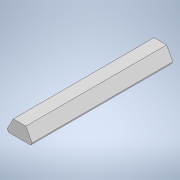
# Autodesk Inventor part: dishHolderArm
Saved by Autodesk Inventor 2022.2 (Build 262287010, 287A)
## iProperties
Created: 2021-09-26
Part Number: dishHolderArm
Material: Generic
Document SubType Name: Modeling
Designer: yiunf
Density: 1 g/cm^3
Appearance: Default
Author: yiunf
## iProperties of the stored document dishHolderArm_3DPrint.ipt
Created: 2021-09-26
Part Number: dishHolderArm_3DPrint
Material: Generic
Document SubType Name: Modeling
Designer: yiunf
Density: 1 g/cm^3
Appearance: Default
Author: yiunf
Autodesk Inventor part; units mm, degrees
ref_plane "YZ Plane" through (0, 0, 0) normal (1, 0, 0) x (0, 1, 0)
ref_plane "XZ Plane" through (0, 0, 0) normal (0, 1, 0) x (-1, 0, 0)
ref_plane "XY Plane" through (0, 0, 0) normal (0, 0, 1) x (1, 0, 0)
sketch "Sketch1" plane through (0, 0, 0) normal (0, 0, 1) x (1, 0, 0)
  line L0 (0, 0) -> (-4.9, 0)
  line L1 (-4.9, 0) -> (4.9, 0)
  line L2 (0, 0) -> (0, 5)
  line L3 (0, 5) -> (-2.5, 5)
  line L4 (-2.5, 5) -> (-4.9, 0)
  line L5 (0, 5) -> (2.5, 5)
  line L6 (2.5, 5) -> (4.9, 0)
  line L7 (0, 0) -> (0, 4)
  line L8 (0, 4) -> (-2.5, 4)
  line L9 (-2.5, 4) -> (-4.9, 0)
  line L10 (0, 4) -> (2.5, 4)
  line L11 (2.5, 4) -> (4.9, 0)
  line L12 (0, 4) -> (0, 5)
  line L13 (0, 4.5) -> (-2.5, 4.5)
  line L14 (-2.5, 4.5) -> (-4.9, 0)
  line L15 (0, 4.5) -> (2.5, 4.5)
  line L16 (2.5, 4.5) -> (4.9, 0)
  line L17 (-4.9, 0) -> (-2.2333, 5)
  line L18 (4.9, 0) -> (2.2333, 5)
  dimension "d0" = 4.9
  dimension "d1" = 9.8
  dimension "d5" = 5
  dimension "d6" = 2.5
  dimension "d7" = 2.5
  dimension "d33" = 4
  constraints: 38 end point, 7 point on line, 3 horizontal, 2 perpendicular, 1 collinear, 1 midpoint, 1 symmetric about line, 1 vertical
  measures "d0" distance of L0.start L0.end
  measures "d1" distance of L0.end L1.end
  measures "d5" distance of L0.start L2.end
  measures "d6" distance of L2.end L3.end
  measures "d7" distance of L2.end L5.end
  measures "d33" distance of L0.start L7.end
extrude "Extrusion1" add sketch "Sketch1" along normal blind 50 contours L2 L10 L11 L1 | L0 L9 L8 L2 | L14 L13 L2 L8 L9 | L11 L10 L2 L15 L16 | L17 L3 L2 L13 | L15 L2 L5 L18
sketch "Sketch2" plane through (0, 0, 50) normal (0, 0, 1) x (1, 0, 0)
  line L0 (0, 5) -> (0, -65)
  circle A0 centre (0, -30) radius 35
  line L1 (-4.9, 0) -> (4.9, 0) projected
  line L2 (4.9, 0) -> (18.0278, 0)
  arc A1 (18.0278, 0) -> (2.5, 5) centre (2.5, -21.6111) ccw
  line L3 (4.9, 0) -> (0, 0)
  line L4 (2.5, 5) -> (0, 5)
  line L5 (-4.9, 0) -> (-18.0278, 0)
  arc A2 (-2.5, 5) -> (-18.0278, 0) centre (-2.5, -21.6111) ccw
  circle A3 centre (0, -30) radius 37.5
  line L6 (2.5, 6.0566) -> (32.476, -11.25)
  line L7 (32.476, -11.25) -> (32.476, -48.75)
  line L8 (32.476, -48.75) -> (0, -67.5)
  line L9 (0, -67.5) -> (-32.476, -48.75)
  line L10 (-32.476, -48.75) -> (-32.476, -11.25)
  line L11 (-32.476, -11.25) -> (-2.5, 6.0566)
  arc A4 (2.5, 6.0566) -> (-2.5, 6.0566) centre (0, 1.7265) ccw
  line L12 (-4.9, 0) -> (-12.9904, 0)
  line L13 (4.9, 0) -> (12.9904, 0)
  line L14 (4.9, 0) -> (-4.9, 0)
  circle A5 centre (0, -30) radius 30
  line L15 (-17.488, -2.5967) -> (0, -30)
  line L16 (0, -30) -> (17.488, -2.5967)
  circle A6 centre (0, -30) radius 32.508
  line L17 (0, -30) -> (-32.476, -11.25)
  line L18 (0, -30) -> (32.476, -11.25)
  arc A7 (-29.976, -9.8066) -> (-32.476, -14.1368) centre (-27.476, -14.1368) ccw
  arc A8 (-32.476, -45.8632) -> (-29.976, -50.1934) centre (-27.476, -45.8632) ccw
  arc A9 (-2.5, -66.0566) -> (2.5, -66.0566) centre (0, -61.7265) ccw
  arc A10 (29.976, -50.1934) -> (32.476, -45.8632) centre (27.476, -45.8632) ccw
  arc A11 (32.476, -14.1368) -> (29.976, -9.8066) centre (27.476, -14.1368) ccw
  line L19 (0, -30) -> (29.976, -9.8066)
  line L20 (2.5, 4.5) -> (-2.5, 4.5) projected
  line L21 (-2.5, 4.5) -> (-4.9, 0)
  line L22 (-2.5, 4.5) -> (-4.9, 0) projected
  line L23 (-4.9, 0) -> (-1.4228, 6.5198)
  point P0 (0, 0)
  point P1 (0, 0)
  point P2 (0, 7.5)
  point P3 (16.1388, -4.7109)
  point P4 (-16.1388, -4.7109)
  point P5 (-1.8396, 6.3758)
  point P6 (25.9808, -15)
  point P7 (-32.4222, -13.4053)
  point P8 (-30.5825, -49.7811)
  point P9 (1.8396, -66.3758)
  point P10 (32.4222, -46.5947)
  point P11 (30.5825, -10.2189)
  point P12 (24.881, -13.2389)
  point P13 (29.976, -9.8066)
  point P14 (-0.9147, 6.6421)
  point P15 (0, 4.5)
  dimension "d13" = 75
  dimension "d14" = 5
  dimension "d28" = 360
  constraints: 42 end point, 26 point on circle, 9 centre point, 7 point on line, 4 coincident, 3 collinear, 3 midpoint, 3 tangent, 2 symmetric about line, 1 vertical, 1 vertical alignment, 53 other
  measures "d14" radius of A4
extrude "Extrusion2" [suppressed]
fillet "Fillet1" [suppressed]
chamfer "Chamfer4" distance 1 angle 45 2 edges at (4.9, 0, 25) (-4.9, 0, 25)
sketch "Sketch4" plane through (0, 0, 50) normal (0, 0, 1) x (1, 0, 0)
  line L0 (-14.1632, 12.0021) -> (30.9274, 12.0021)
  line L1 (30.9274, 12.0021) -> (30.9274, -18.7889)
  line L2 (30.9274, -18.7889) -> (-14.1632, -18.7889)
  line L3 (-14.1632, -18.7889) -> (-14.1632, 12.0021)
  line L4 (-3.9, 0) -> (-4.4294, 0.8824) projected
  line L5 (-3.9, 0) -> (-4.4294, 0.8824)
  line L6 (-2.5, 4.5) -> (-4.4294, 0.8824) projected
  line L7 (-4.4294, 0.8824) -> (-2.5, 4.5)
  line L8 (2.5, 4.5) -> (-2.5, 4.5) projected
  line L9 (-2.5, 4.5) -> (2.5, 4.5)
  line L10 (-3.9, 0) -> (0, 0) projected
  line L11 (3.9, 0) -> (-3.9, 0)
  line L12 (3.9, 0) -> (4.4294, 0.8824) projected
  line L13 (3.9, 0) -> (4.4294, 0.8824)
  line L14 (4.4294, 0.8824) -> (2.5, 4.5) projected
  line L15 (4.4294, 0.8824) -> (2.5, 4.5)
  line L16 (2.2333, 5) -> (4.4294, 0.8824) projected
  line L17 (-2.2333, 5) -> (2.2333, 5) projected
  line L18 (-1.4228, 6.5198) -> (-4.4294, 0.8824) projected
  constraints: 20 end point, 6 collinear, 2 parallel, 1 horizontal, 1 perpendicular
extrude "Extrusion3" cut sketch "Sketch4" against normal blind 7.5
body "Solid1"
